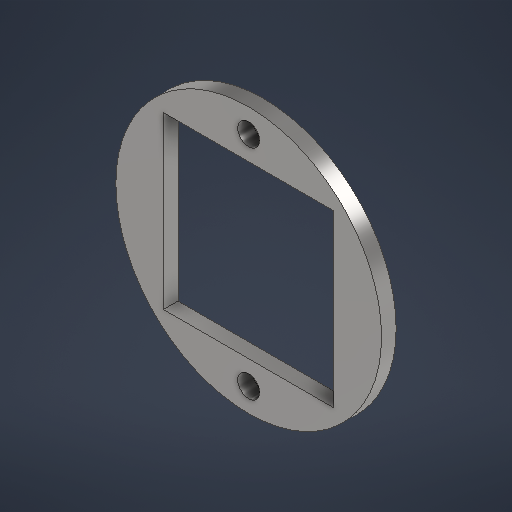
# Autodesk Inventor part: Part3_A_Y
Saved by Autodesk Inventor 2026 (Build 300175050, 175E)
## iProperties
Created: 2026-01-08
Part Number: Part3_A_Y
Material: 鋼、軟鋼
Document SubType Name: Modeling
Designer: Kota-Inoue
Density: 7.85 g/cm^3
Appearance: 半つや出し
Mass: 641.479 g
Surface Area: 319.402 cm^2
Volume: 81.7171 cm^3
Author: Kota-Inoue
Autodesk Inventor part; units mm, degrees
ref_plane "YZ Plane" through (0, 0, 0) normal (1, 0, 0) x (0, 1, 0)
ref_plane "XZ Plane" through (0, 0, 0) normal (0, 1, 0) x (-1, 0, 0)
ref_plane "XY Plane" through (0, 0, 0) normal (0, 0, 1) x (1, 0, 0)
sketch "スケッチ1" plane through (0, 0, 0) normal (0, 0, 1) x (1, 0, 0)
  circle A0 centre (0, 0) radius 27.25
  line L0 (17.5, 17.5) -> (-17.5, 17.5)
  line L1 (-17.5, 17.5) -> (-17.5, -17.5)
  line L2 (-17.5, -17.5) -> (17.5, -17.5)
  line L3 (17.5, -17.5) -> (17.5, 17.5)
  line L4 (17.5, 17.5) -> (-17.5, -17.5) construction
  line L5 (-17.5, 17.5) -> (17.5, -17.5) construction
  line L6 (1, 17.5) -> (-1, 17.5)
  line L7 (-1, -17.5) -> (1, -17.5)
  dimension "d0" = 54.5
  dimension "d6" = 35
  dimension "d107" = 2
  dimension "d108" = 35
  constraints: 16 end point, 3 parallel, 2 horizontal, 2 midpoint, 2 perpendicular, 1 centre point, 1 coincident
  measures "d0" diameter of A0
  measures "d6" distance of L0.start L0.end
  measures "d107" distance of L7.end L7.start
  measures "d108" distance of L7.start L6.end
extrude "押し出し1" add sketch "スケッチ1" against normal blind 3
sketch "スケッチ8" plane through (0, 0, 0) normal (0, 0, 1) x (1, 0, 0)
  circle A0 centre (0, 0) radius 27.25
  circle A1 centre (0, 0) radius 22.375
  line L0 (0, 30.4962) -> (0, -31.0616)
  point P0 (0, 0)
  point P1 (0, 22.375)
  point P2 (0, -22.375)
  dimension "d111" = 44.75
  dimension "d112" = 54.5
  constraints: 2 centre point, 2 coincident, 2 end point, 2 point on circle, 2 point on line, 1 vertical
  measures "d111" diameter of A1
  measures "d112" diameter of A0
hole "穴5" at (0, 22.375, 0) at (0, -22.375, 0) direction (0, 0, -1) diameter 4.5 end through all clearance for "Countersunk Flat Head Screw ISO 2009/7046" size "M4" standard "ISO"
